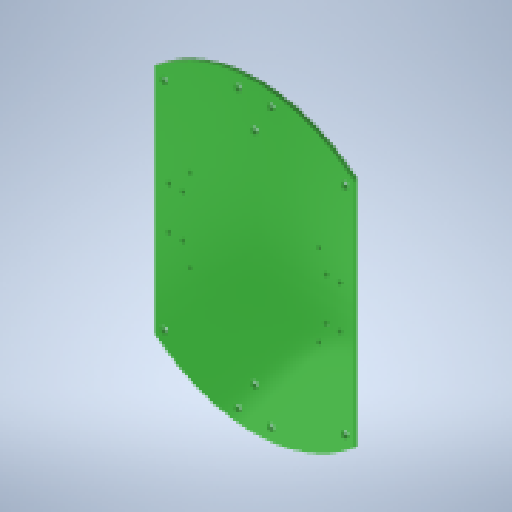
# Autodesk Inventor part: BaseBoard2
Saved by Autodesk Inventor 2025.3 (Build 293356000, 356)
## iProperties
Created: 2025-05-29
Part Number: BaseBoard2
Material: 一般
Document SubType Name: Modeling
Designer: yamashita1
Density: 1 g/cm^3
Appearance: 滑らか - 濃い深緑
Author: yamashita1
Autodesk Inventor part; units mm, degrees
ref_plane "YZ Plane" through (0, 0, 0) normal (1, 0, 0) x (0, 1, 0)
ref_plane "XZ Plane" through (0, 0, 0) normal (0, 1, 0) x (-1, 0, 0)
ref_plane "XY Plane" through (0, 0, 0) normal (0, 0, 1) x (1, 0, 0)
sketch "スケッチ1" plane through (0, 0, 0) normal (0, 0, 1) x (1, 0, 0)
  circle A0 centre (0, 0) radius 65 construction
  line L0 (-42.5, 65) -> (42.5, 65) construction
  line L1 (42.5, 65) -> (42.5, -65) construction
  line L2 (42.5, -65) -> (-42.5, -65) construction
  line L3 (-42.5, -65) -> (-42.5, 65) construction
  arc A1 (42.5, 49.1808) -> (-42.5, 49.1808) centre (0, 0) ccw
  line L4 (-42.5, 49.1808) -> (-42.5, -49.1808)
  line L5 (42.5, 49.1808) -> (42.5, -49.1808)
  arc A2 (-42.5, -49.1808) -> (42.5, -49.1808) centre (0, 0) ccw
  point P0 (0, 65)
  dimension "d0" = 130
  dimension "d1" = 85
  constraints: 14 end point, 9 point on circle, 4 point on line, 3 centre point, 3 parallel, 2 tangent, 1 coincident, 1 concentric, 1 horizontal, 1 midpoint, 1 perpendicular, 1 vertical, 1 vertical alignment
  measures "d0" diameter of A0
  measures "d1" distance of L1.end L2.end
extrude "基板" add sketch "スケッチ1" along normal blind 1.6
sketch "スケッチ2" plane through (0, 0, 1.6) normal (0, 0, 1) x (1, 0, 0)
  line L0 (-100.8621, 0) -> (100.8621, 0) construction
  line L1 (0, 110.7931) -> (0, -110.7931) construction
  line L2 (-42.5, 49.1808) -> (-42.5, -49.1808) construction
  circle A0 centre (0, 0) radius 60 construction
  point P0 (-36.5, 9)
  point P1 (-30.5, 9)
  point P2 (30.5, 9)
  point P3 (36.5, 9)
  point P4 (-36.5, -9)
  point P5 (-30.5, -9)
  point P6 (30.5, -9)
  point P7 (36.5, -9)
  point P8 (-40, -30)
  point P9 (-40, -45)
  point P10 (-42.5, -49.1808)
  point P11 (-27.5, -17.5)
  point P12 (-27.5, 17.5)
  point P13 (27.5, -17.5)
  point P14 (27.5, 17.5)
  dimension "d4" = 18
  dimension "d5" = 6
  dimension "d6" = 6
  dimension "d26" = 120
  dimension "d38" = 35
  dimension "d39" = 15
  constraints: 8 horizontal alignment, 5 symmetric about line, 5 vertical alignment, 4 end point, 3 coincident, 3 midpoint, 1 centre point, 1 horizontal, 1 vertical, 1 other
  measures "d4" distance of point (-36.5, -9) point (-36.5, 9)
  measures "d6" distance of point (-30.5, 9) point (-36.5, 9)
  measures "d26" diameter of A0
  measures "d38" distance of point (-27.5, 17.5) point (-27.5, -17.5)
hole "モータ取付穴" at (-36.5, 9, 1.6) at (-30.5, 9, 1.6) at (30.5, 9, 1.6) at (36.5, 9, 1.6) at (-36.5, -9, 1.6) at (-30.5, -9, 1.6) at (30.5, -9, 1.6) at (36.5, -9, 1.6) at (-27.5, -17.5, 1.6) at (-27.5, 17.5, 1.6) at (27.5, -17.5, 1.6) at (27.5, 17.5, 1.6) direction (0, 0, -1) diameter 2.1 end through all
sketch "スケッチ3" plane through (0, 0, 1.6) normal (0, 0, 1) x (1, 0, 0)
  line L0 (0, 0) -> (0, 55.332) construction
  line L1 (-15.38, 55) -> (15.38, 55) construction
  line L2 (0, 46.85) -> (-7.0581, 50.925) construction
  line L3 (-7.0581, 50.925) -> (-7.0581, 59.075) construction
  line L4 (-7.0581, 59.075) -> (0, 63.15) construction
  line L5 (0, 63.15) -> (7.0581, 59.075) construction
  line L6 (7.0581, 59.075) -> (7.0581, 50.925) construction
  line L7 (7.0581, 50.925) -> (0, 46.85) construction
  arc A0 (42.5, 49.1808) -> (-42.5, 49.1808) centre (0, 0) ccw construction
  point P0 (0, 55)
  point P1 (0, 55)
  point P2 (0, 65)
  dimension "d17" = 16.3
  dimension "d18" = 10
  constraints: 16 end point, 7 coincident, 2 point on line, 1 horizontal, 1 midpoint, 1 point on circle, 1 vertical, 13 other
  measures "d17" distance of L2.start L4.end
  measures "d18" distance from line of point (0, 65) L1
hole "ボールキャスター取付穴" at (-7.0581, 59.075, 1.6) at (7.0581, 59.075, 1.6) at (0, 46.85, 1.6) direction (0, 0, -1) diameter 3.2 end through all
sketch "スケッチ4" plane through (0, 0, 1.6) normal (0, 0, 1) x (1, 0, 0)
  line L0 (0, -55.1622) -> (0, 55.1622) construction
  line L1 (42.5, -49.1808) -> (42.5, 49.1808) construction
  circle A0 centre (0, 0) radius 60 construction
  line L2 (0, 0) -> (36.3616, 43.334) construction
  line L3 (0, 0) -> (56.5685, 0) construction
  point P0 (38.5, -46.019)
  point P1 (-38.5, -46.019)
  point P2 (38.5673, 45.9627)
  point P3 (-38.5673, 45.9627)
  dimension "d27" = 4
  dimension "d29" = 120
  dimension "d30" = 50
  constraints: 6 end point, 2 coincident, 2 point on circle, 2 symmetric about line, 1 centre point, 1 equal length, 1 horizontal, 1 midpoint, 1 point on line, 1 vertical
  measures "d27" distance from line of L1 A0.end
  measures "d29" diameter of A0
  measures "d30" angle of L3 L2
hole "スペーサ取付穴" at (38.5, -46.019, 1.6) at (-38.5, -46.019, 1.6) at (38.5673, 45.9627, 1.6) at (-38.5673, 45.9627, 1.6) direction (0, 0, -1) diameter 3.2 end through all
mirror "ミラー1" about plane through (0, 0, 0) normal (0, 1, 0) of "ボールキャスター取付穴"
